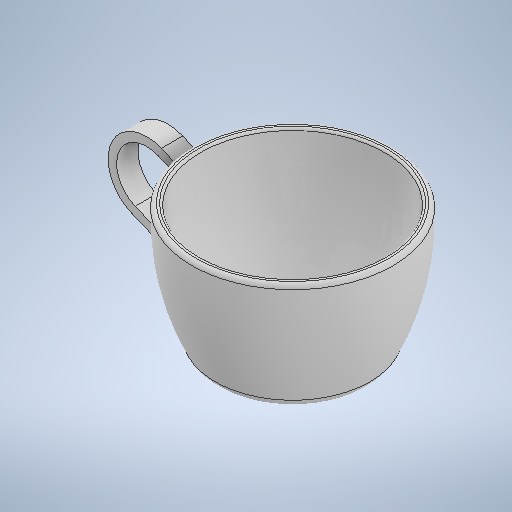
# Autodesk Inventor part: cad@48
Saved by Autodesk Inventor 2025.2 (Build 292293000, 293)
## iProperties
Created: 2025-04-05
Part Number: cad@48
Material: Generic
Document SubType Name: Modeling
Designer: spars
Density: 1 g/cm^3
Appearance: Default
Author: spars
Autodesk Inventor part; units mm, degrees
ref_plane "YZ Plane" through (0, 0, 0) normal (1, 0, 0) x (0, 1, 0)
ref_plane "XZ Plane" through (0, 0, 0) normal (0, 1, 0) x (-1, 0, 0)
ref_plane "XY Plane" through (0, 0, 0) normal (0, 0, 1) x (1, 0, 0)
sketch "Sketch1" plane through (0, 0, 0) normal (0, 0, 1) x (1, 0, 0)
  line L0 (0, 0) -> (-14.8816, 0)
  arc A0 (-21.4937, 27.4816) -> (-15.7787, 0.5583) centre (34.4634, 25.2915) ccw
  line L1 (-13.5966, -2.0522) -> (0, -2.0522)
  arc A1 (-23.5105, 27.0312) -> (-18.1305, 0.8399) centre (34.4634, 25.2915) ccw
  line L2 (-21.9934, 28.0012) -> (-22.5109, 28.0012)
  arc A2 (-22.5109, 28.0012) -> (-23.5105, 27.0312) centre (-22.5109, 27.0012) ccw
  arc A3 (-21.4937, 27.4816) -> (-21.9934, 28.0012) centre (-21.9934, 27.5012) ccw
  arc A4 (-15.7787, 0.5583) -> (-14.8816, 0) centre (-14.8816, 1) ccw
  arc A5 (-18.1305, 0.8399) -> (-13.5966, -2.0522) centre (-13.5966, 2.9478) ccw
  line L3 (0, 0) -> (0, -2.0522)
  line L4 (0, 36.6448) -> (0, -24.0001)
  point P0 (-15.5, 0)
  point P1 (-16.6866, -2.0522)
  point P2 (-23.4733, 28.0012)
  dimension "d6" = 15.5
  dimension "d9" = 56
  dimension "d10" = 2
  dimension "d11" = 1
  dimension "d12" = 1
  dimension "d13" = 1
  dimension "d14" = 5
  constraints: 15 point on circle, 10 end point, 8 tangent, 6 centre point, 3 point on line, 2 horizontal, 1 perpendicular, 1 vertical
  measures "d6" distance of L0.start point (-15.5, 0)
  measures "d9" radius of A0
  measures "d10" radial gap between concentric circles of A0 A1
  measures "d11" radius of A2
  measures "d12" diameter of A3
  measures "d13" radius of A4
  measures "d14" radius of A5
revolve "Revolution1" add sketch "Sketch1" angle 360 mid plane about axis through (0, 36.6448, 0) along (0, -1, 0)
sketch "Sketch2" plane through (0, 0, 0) normal (0, 0, 1) x (1, 0, 0)
  line L0 (-38.1062, 20.566) -> (-23.6454, 14.5878) construction
  line L1 (-34.3116, 11.4227) -> (-26.4836, 8.1866)
  line L2 (-23.4477, 22.0807) -> (-28.9629, 24.3607)
  arc A0 (-28.9629, 24.3607) -> (-34.3116, 11.4227) centre (-31.6372, 17.8917) ccw
  line L3 (-26.4836, 8.1866) -> (-19.9554, 5.2268)
  arc A1 (-23.5105, 27.0312) -> (-18.1305, 0.8399) centre (34.4634, 25.2915) ccw projected
  line L4 (-35.0756, 9.5744) -> (-27.2788, 6.3511)
  line L5 (-27.2788, 6.3511) -> (-18.8916, 2.5486)
  line L6 (-23.5277, 24.2779) -> (-28.1988, 26.209)
  arc A2 (-28.1988, 26.209) -> (-35.0756, 9.5744) centre (-31.6372, 17.8917) ccw
  arc A3 (-23.4477, 22.0807) -> (-23.416, 21.554) centre (34.4634, 25.2915) ccw
  arc A4 (-23.5277, 24.2779) -> (-23.4477, 22.0807) centre (34.4634, 25.2915) ccw
  arc A5 (-23.5277, 24.2779) -> (-23.4477, 22.0807) centre (34.4634, 25.2915) ccw
  line L7 (-18.8916, 2.5486) -> (-19.9554, 5.2268)
  point P0 (0, 0)
  point P1 (-30.8758, 17.5769)
  dimension "d19" = 2
  constraints: 18 end point, 16 point on circle, 5 centre point, 2 parallel, 2 tangent, 1 concentric, 1 midpoint
  measures "d19" radial gap between concentric circles of A0 A2
extrude "Extrusion1" add sketch "Sketch2" along normal mid plane 5 contours L1 L3 A1 L5 L4 A2 L6 L2 A0
body "Solid1"
